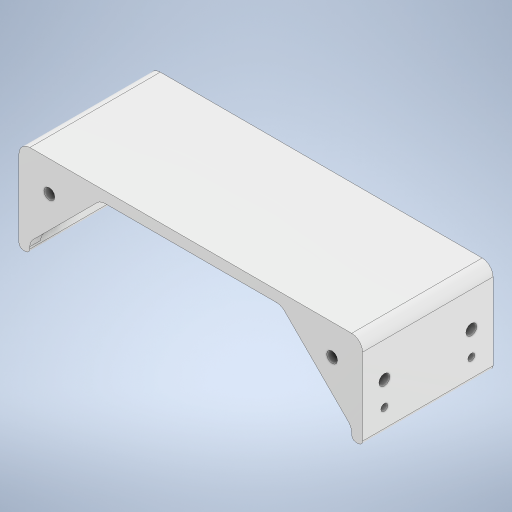
# Autodesk Inventor part: BP_BOX-60
Saved by Autodesk Inventor 2024.3 (Build 283343000, 343)
## iProperties
Created: 2025-10-30
Part Number: BP_BOX-60
Material: ABS プラスチック
Document SubType Name: Modeling
Designer: 佐藤智貴
Density: 1.06 g/cm^3
Appearance: 滑らか - 白
Mass: 64.4893 g
Surface Area: 354.929 cm^2
Volume: 60.8389 cm^3
Author: 佐藤智貴
Autodesk Inventor part; units mm, degrees
ref_plane "YZ Plane" through (0, 0, 0) normal (1, 0, 0) x (0, 1, 0)
ref_plane "XZ Plane" through (0, 0, 0) normal (0, 1, 0) x (-1, 0, 0)
ref_plane "XY Plane" through (0, 0, 0) normal (0, 0, 1) x (1, 0, 0)
sketch "スケッチ1" plane through (0, 0, 0) normal (0, 0, 1) x (1, 0, 0)
  line L0 (0, 0) -> (158, 0)
  line L1 (158, 0) -> (158, 250)
  line L2 (158, 250) -> (0, 250)
  line L3 (0, 250) -> (0, 0)
  line L4 (5, 245) -> (153, 245)
  line L5 (153, 245) -> (153, 5)
  line L6 (153, 5) -> (5, 5)
  line L7 (5, 5) -> (5, 245)
  line L8 (79, 250) -> (79, 0)
  line L9 (0, 125) -> (158, 125)
  line L10 (0, 245) -> (158, 245)
  line L11 (158, 245) -> (158, 3)
  line L12 (158, 3) -> (0, 3)
  line L13 (0, 3) -> (0, 245)
  point P0 (158, 245)
  point P1 (0, 3)
  point P2 (79, 3)
  point P3 (79, 5)
  point P4 (5, 125)
  point P5 (153, 125)
  point P6 (79, 245)
  point P7 (79, 245)
  point P8 (79, 125)
  point P9 (0, 3)
  dimension "d0" = 158
  dimension "d1" = 250
  dimension "d2" = 5
  dimension "d73" = 5
  constraints: 28 end point, 6 parallel, 4 midpoint, 3 perpendicular, 2 horizontal, 2 point on line, 3 other
  measures "d0" distance of L1.end L2.end
  measures "d1" distance between parallel lines of L0 L2
  measures "d2" distance between parallel lines of L2 L4
  measures "d73" distance between parallel lines of L2 L10
extrude "押し出し1" add sketch "スケッチ1" along normal blind 60 contours L3 L2 L8 L4 L10 | L10 L4 L8 L2 L1
sketch "スケッチ5" plane through (0, 0, 0) normal (0, 0, -1) x (-1, 0, 0)
  line L0 (0, 250) -> (0, 0) projected
  line L1 (0, 250) -> (-50, 250)
  line L2 (-50, 250) -> (-50, 200)
  line L3 (-50, 200) -> (0, 200)
  line L4 (0, 200) -> (0, 250)
  line L5 (-50, 250) -> (0, 200)
  line L6 (-46.2132, 253.7868) -> (3.7868, 203.7868)
  line L7 (0, 0) -> (-158, 0) projected
  line L8 (0, 125) -> (-79, 125)
  line L9 (-79, 125) -> (-79, 0)
  line L10 (-79, 0) -> (0, 0)
  line L11 (0, 0) -> (0, 125)
  line L12 (-46.2132, -3.7868) -> (3.7868, 46.2132)
  line L13 (-111.7868, 253.7868) -> (-161.7868, 203.7868)
  line L14 (-111.7868, -3.7868) -> (-161.7868, 46.2132)
  line L15 (0, 0) -> (-50, 0)
  line L16 (0, 50) -> (0, 0)
  line L17 (-158, 250) -> (-158, 0)
  line L18 (-158, 0) -> (0, 0)
  line L19 (-158, 250) -> (-108, 250)
  point P0 (0, 42.4264)
  point P1 (-42.4264, 0)
  point P2 (-158, 42.4264)
  point P3 (-115.5736, 0)
  point P4 (-42.4264, 250)
  point P5 (0, 207.5736)
  point P6 (-115.5736, 250)
  point P7 (-158, 207.5736)
  dimension "d29" = 50
  dimension "d30" = 50
  dimension "d31" = 30
  constraints: 36 end point, 12 symmetric about line, 5 parallel, 2 horizontal, 2 midpoint, 2 perpendicular
  measures "d29" distance of L2.end L3.end
  measures "d30" distance of L1.end L2.end
  measures "d31" distance from line of L0.start L6
extrude "押し出し3" add sketch "スケッチ5" against normal blind 5 contours L0 L6 L1 | L13 L17 L19
sketch "スケッチ6" plane through (0, 0, 60) normal (0, 0, 1) x (1, 0, 0)
  line L0 (0, 0) -> (50, 0)
  line L1 (50, 0) -> (50, 50)
  line L2 (50, 50) -> (0, 50)
  line L3 (0, 50) -> (0, 0)
  line L4 (50, 0) -> (0, 50)
  line L5 (46.2132, -3.7868) -> (-3.7868, 46.2132)
  line L6 (0, 250) -> (0, 0) projected
  line L7 (158, 250) -> (0, 250) projected
  line L8 (0, 125) -> (79, 125)
  line L9 (79, 125) -> (79, 250)
  line L10 (79, 250) -> (0, 250)
  line L11 (0, 250) -> (0, 125)
  line L12 (0, 250) -> (50, 250)
  line L13 (0, 200) -> (0, 250)
  line L14 (46.2132, 253.7868) -> (-3.7868, 203.7868)
  line L15 (158, 0) -> (108, 0)
  line L16 (158, 50) -> (158, 0)
  line L17 (111.7868, -3.7868) -> (161.7868, 46.2132)
  line L18 (158, 250) -> (158, 0)
  line L19 (158, 250) -> (108, 250)
  line L20 (111.7868, 253.7868) -> (161.7868, 203.7868)
  point P0 (158, 42.4264)
  point P1 (115.5736, 0)
  point P2 (158, 207.5736)
  point P3 (115.5736, 250)
  point P4 (0, 207.5736)
  point P5 (42.4264, 250)
  point P6 (42.4264, 0)
  point P7 (0, 42.4264)
  dimension "d34" = 50
  dimension "d35" = 50
  dimension "d37" = 30
  constraints: 38 end point, 14 symmetric about line, 5 parallel, 2 horizontal, 2 midpoint, 2 perpendicular
  measures "d34" distance of L1.end L2.end
  measures "d35" distance of L0.end L1.end
  measures "d37" distance from line of L5 L0.start
extrude "押し出し4" add sketch "スケッチ6" against normal blind 5 contours L6 L7 L14 | L18 L20 L7
sketch "スケッチ7" plane through (0, 0, 0) normal (0, 0, -1) x (-1, 0, 0)
  line L0 (0, 0) -> (-158, 0) projected
  line L1 (0, 124.7294) -> (-79, 124.7294)
  line L2 (-79, 124.7294) -> (-79, 0)
  line L3 (-79, 0) -> (0, 0)
  line L4 (0, 0) -> (0, 124.7294)
  line L5 (0, 250) -> (0, 0) projected
  line L6 (-158, 250) -> (0, 250) projected
  point P0 (-14, 236)
  point P1 (-14, 13.4587)
  point P2 (-144, 236)
  point P3 (-144, 13.4587)
  point P4 (0, 207.5736)
  dimension "d70" = 130
  dimension "d71" = 14
  dimension "d72" = 14
  constraints: 8 end point, 3 symmetric about line, 2 parallel, 1 horizontal, 1 midpoint, 1 perpendicular
  measures "d70" distance of point (-144, 236) point (-14, 236)
  measures "d71" distance from line of L5 point (-14, 236)
  measures "d72" distance from line of L6 point (-144, 236)
hole "穴2" at (14, 236, 0) at (14, 13.4587, 0) at (144, 236, 0) at (144, 13.4587, 0) direction (0, 0, 1) diameter 5 end through all
sketch "スケッチ8" plane through (158, 250, 60) normal (1, 0, 0) x (0, 0, -1)
  line L0 (60, 0) -> (0, 0) projected
  line L1 (60, -42.4264) -> (55, -42.4264) projected
  line L2 (0, 0) -> (60, 0)
  line L3 (60, 0) -> (60, -42.4264)
  line L4 (60, -42.4264) -> (0, -42.4264)
  line L5 (0, -42.4264) -> (0, 0)
  point P0 (60, -250)
  constraints: 8 end point, 2 parallel, 1 horizontal, 1 perpendicular
extrude "押し出し5" add sketch "スケッチ8" against normal blind 5
sketch "スケッチ9" plane through (0, 250, 0) normal (-1, 0, 0) x (0, 0, 1)
  line L0 (60, 0) -> (60, -42.4264) projected
  line L1 (0, 0) -> (0, -250) projected
  line L2 (60, 0) -> (0, 0)
  line L3 (0, 0) -> (0, -42.4264)
  line L4 (0, -42.4264) -> (60, -42.4264)
  line L5 (60, -42.4264) -> (60, 0)
  point P0 (60, -250)
  constraints: 8 end point, 2 parallel, 1 horizontal, 1 perpendicular
extrude "押し出し6" add sketch "スケッチ9" against normal blind 5
sketch "スケッチ10" plane through (0, 250, 0) normal (-1, 0, 0) x (0, 0, 1)
  line L0 (55, -37.4264) -> (55, -5) projected
  line L1 (0, -37.4264) -> (5, -37.4264) projected
  line L2 (55, -5) -> (5, -5)
  line L3 (5, -5) -> (5, -37.4264)
  line L4 (5, -37.4264) -> (55, -37.4264)
  line L5 (55, -37.4264) -> (55, -5)
  line L6 (60, 0) -> (60, -42.4264) projected
  line L7 (60, -42.4264) -> (0, -42.4264)
  line L8 (0, -42.4264) -> (0, -37.4264)
  line L9 (0, -37.4264) -> (60, -37.4264)
  line L10 (60, -37.4264) -> (60, -42.4264)
  circle A0 centre (50, -21) radius 2.5
  circle A1 centre (10, -21) radius 2.5
  circle A2 centre (50, -32) radius 1.6
  circle A3 centre (10, -32) radius 1.6
  line L11 (0, 0) -> (0, -250) projected
  line L12 (0, 0) -> (60, 0) projected
  point P0 (-5.1594, -27.8126)
  point P1 (60, -250)
  dimension "d55" = 5
  dimension "d56" = 5
  dimension "d57" = 40
  dimension "d58" = 10
  dimension "d63" = 3.2
  dimension "d64" = 3.2
  dimension "d65" = 40
  dimension "d66" = 11
  dimension "d67" = 11
  dimension "d68" = 10
  dimension "d74" = 21
  dimension "d75" = 21
  constraints: 16 end point, 4 centre point, 4 parallel, 2 horizontal, 2 perpendicular
  measures "d55" diameter of A0
  measures "d56" diameter of A1
  measures "d57" distance of A0.centre A1.centre
  measures "d58" distance from line of L6 A0.centre
  measures "d63" diameter of A2
  measures "d64" diameter of A3
  measures "d65" distance of A2.centre A3.centre
  measures "d66" distance of A0.centre A2.centre
  measures "d67" distance of A1.centre A3.centre
  measures "d68" distance from line of L11 A3.centre
  measures "d74" distance from line of L12 A0.centre
  measures "d75" distance from line of L12 A1.centre
extrude "押し出し7" cut sketch "スケッチ10" against normal through all contours A0 | A1 | A2 | A3
fillet "フィレット4" radius 5 12 edges at (0, 250, 30) (158, 250, 30) (120.5736, 245, 57.5) (120.5736, 245, 2.5) (153, 245, 30) (5, 245, 30) (37.4264, 245, 57.5) (37.4264, 245, 2.5) (153, 212.5736, 2.5) (153, 212.5736, 57.5) (5, 212.5736, 2.5) (5, 212.5736, 57.5)
fillet "フィレット6" radius 2 4 edges at (153, 207.5736, 30) (0, 207.5736, 30) (5, 207.5736, 30) (158, 207.5736, 30)
sketch "スケッチ12" plane through (37.4264, 245, 0) normal (0, -1, 0) x (1, 0, 0)
  line L0 (-27.4264, 5) -> (2.0711, 5) projected
  line L1 (2.0711, 0) -> (81.0761, 0) projected
  line L2 (81.0761, 5) -> (110.5736, 5) projected
  line L3 (110.5736, 55) -> (81.0761, 55) projected
  line L4 (2.0711, 60) -> (81.0761, 60) projected
  line L5 (2.0711, 55) -> (-27.4264, 55) projected
  line L6 (78.1472, 55) -> (78.1472, 50)
  line L7 (78.1472, 50) -> (108.5736, 50)
  line L8 (108.5736, 50) -> (108.5736, 10)
  line L9 (108.5736, 10) -> (76.1819, 10)
  line L10 (76.1819, 10) -> (76.1819, 5)
  line L11 (76.1819, 5) -> (3.0347, 5)
  line L12 (3.0347, 5) -> (3.0347, 10)
  line L13 (3.0347, 10) -> (-25.4264, 10)
  line L14 (-25.4264, 10) -> (-25.4264, 50)
  line L15 (-25.4264, 50) -> (3.0347, 50)
  line L16 (3.0347, 50) -> (3.0347, 55)
  line L17 (3.0347, 55) -> (78.1472, 55)
  line L18 (2.0711, 0) -> (2.0711, 5) projected
  line L19 (81.0761, 5) -> (81.0761, 0) projected
  line L20 (110.5736, 55) -> (110.5736, 5) projected
  line L21 (81.0761, 60) -> (81.0761, 55) projected
  line L22 (2.0711, 55) -> (2.0711, 60) projected
  line L23 (-27.4264, 5) -> (-27.4264, 55) projected
  line L24 (115.5736, 60) -> (115.5736, 0) projected
  line L25 (-32.4264, 0) -> (-32.4264, 60) projected
  point P0 (-37.4264, 0)
  dimension "d76" = 5
  dimension "d81" = 7
  dimension "d82" = 5
  dimension "d83" = 40
  dimension "d84" = 7
  constraints: 24 end point
  measures "d76" distance between parallel lines of L4 L17
  measures "d81" distance between parallel lines of L24 L8
  measures "d82" distance between parallel lines of L25 L23
  measures "d83" distance of L13.end L14.end
  measures "d84" distance between parallel lines of L25 L14
extrude "押し出し8" cut sketch "スケッチ12" against normal blind 3 contours L6 L7 L8 L9 L10 L11 L12 L13 L14 L15 L16 L17
fillet "フィレット7" radius 2 12 edges at (146, 246.5, 10) (146, 246.5, 50) (115.5736, 246.5, 50) (113.6083, 246.5, 10) (115.5736, 246.5, 55) (113.6083, 246.5, 5) (40.4611, 246.5, 5) (40.4611, 246.5, 10) (12, 246.5, 10) (40.4611, 246.5, 55) (40.4611, 246.5, 50) (12, 246.5, 50)
equation "\"d35\" = d34"
equation "\"d56\" = d55"
equation "\"d63\" = d64"
equation "\"d67\" = d66"
